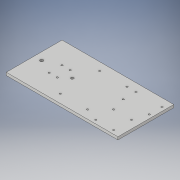
# Autodesk Inventor part: BaseBoard
Saved by Autodesk Inventor 2017 (Build 210142000, 142)
## iProperties
Created: 2016-11-29
Part Number: BaseBoard
Material: Generic
Document SubType Name: Modeling
Designer: Mark
Density: 1 g/cm^3
Appearance: Default
Author: Mark
Autodesk Inventor part; units mm, degrees
ref_plane "YZ Plane" through (0, 0, 0) normal (1, 0, 0) x (0, 1, 0)
ref_plane "XZ Plane" through (0, 0, 0) normal (0, 1, 0) x (-1, 0, 0)
ref_plane "XY Plane" through (0, 0, 0) normal (0, 0, 1) x (1, 0, 0)
sketch "Sketch1" plane through (0, 0, 0) normal (0, 1, 0) x (-1, 0, 0)
  line L0 (0, 0) -> (254, 0)
  line L1 (254, 0) -> (254, -127)
  line L2 (254, -127) -> (0, -127)
  line L3 (0, -127) -> (0, 0)
  circle A0 centre (17.9672, -8.2233) radius 1.905
  circle A1 centre (17.9672, -48.8633) radius 1.905
  circle A2 centre (58.6072, -48.8633) radius 1.905
  circle A3 centre (58.6072, -8.2233) radius 1.905
  circle A4 centre (67.644, -79.6665) radius 1.905
  circle A5 centre (67.644, -108.6225) radius 1.905
  circle A6 centre (8.462, -79.6665) radius 1.905
  circle A7 centre (8.462, -108.6225) radius 1.905
  circle A8 centre (236.9221, -63.5) radius 3.81
  circle A9 centre (167.3261, -63.5) radius 3.175
  circle A10 centre (150.3735, -19.2274) radius 1.905
  circle A11 centre (150.3735, -108.8774) radius 1.905
  circle A12 centre (88.1435, -108.8774) radius 1.905
  circle A13 centre (88.1435, -19.2274) radius 1.905
  circle A14 centre (204.3299, -47.9) radius 1.905
  circle A15 centre (204.3299, -77.11) radius 1.905
  circle A16 centre (185.7625, -77.11) radius 1.905
  circle A17 centre (185.7625, -47.9) radius 1.905
  dimension "d0" = 254
  dimension "d1" = 127
  dimension "d2" = 3.81
  dimension "d3" = 3.81
  dimension "d4" = 3.81
  dimension "d5" = 3.81
  dimension "d6" = 40.64
  dimension "d7" = 40.64
  dimension "d8" = 40.64
  dimension "d9" = 40.64
  dimension "d14" = 3.81
  dimension "d15" = 3.81
  dimension "d16" = 3.81
  dimension "d17" = 3.81
  dimension "d18" = 7.62
  dimension "d19" = 63.5
  dimension "d20" = 6.35
  dimension "d21" = 69.596
  dimension "d22" = 63.5
  dimension "d25" = 3.81
  dimension "d26" = 3.81
  dimension "d27" = 3.81
  dimension "d28" = 3.81
  dimension "d31" = 3.81
  dimension "d32" = 3.81
  dimension "d33" = 3.81
  dimension "d34" = 3.81
  constraints: 18 centre point, 8 end point, 2 parallel, 1 horizontal, 1 perpendicular
  measures "d0" distance of L1.end L2.end
  measures "d1" distance of L0.end L1.end
  measures "d2" diameter of A0
  measures "d3" diameter of A1
  measures "d4" diameter of A2
  measures "d5" diameter of A3
  measures "d6" distance of A1.centre A0.centre
  measures "d7" distance of A3.centre A0.centre
  measures "d8" distance of A2.centre A3.centre
  measures "d9" distance of A1.centre A2.centre
  measures "d14" diameter of A4
  measures "d15" diameter of A5
  measures "d16" diameter of A6
  measures "d17" diameter of A7
  measures "d18" diameter of A8
  measures "d19" distance from line of L2 A8.centre
  measures "d20" diameter of A9
  measures "d21" distance of A9.centre A8.centre
  measures "d22" distance from line of L2 A9.centre
  measures "d25" diameter of A10
  measures "d26" diameter of A11
  measures "d27" diameter of A12
  measures "d28" diameter of A13
  measures "d31" diameter of A14
  measures "d32" diameter of A15
  measures "d33" diameter of A16
  measures "d34" diameter of A17
extrude "Extrusion1" add sketch "Sketch1" along normal blind 6.35
body "Solid1"
